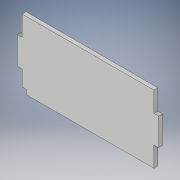
# Autodesk Inventor part: lower_front_wall
Saved by Autodesk Inventor 2018 (Build 220112000, 112)
## iProperties
Created: 2018-04-09
Part Number: lower_front_wall
Material: Generic
Document SubType Name: Modeling
Designer: guita
Density: 1 g/cm^3
Appearance: Default
Author: guita
Autodesk Inventor part; units mm, degrees
ref_plane "YZ Plane" through (0, 0, 0) normal (1, 0, 0) x (0, 1, 0)
ref_plane "XZ Plane" through (0, 0, 0) normal (0, 1, 0) x (-1, 0, 0)
ref_plane "XY Plane" through (0, 0, 0) normal (0, 0, 1) x (1, 0, 0)
sketch "Sketch1" plane through (0, 0, 0) normal (0, 0, 1) x (1, 0, 0)
  line L0 (0, 0) -> (184.15, 0)
  line L1 (184.15, 94.488) -> (0, 94.488)
  line L2 (190.5, 47.244) -> (190.5, 66.294)
  line L3 (190.5, 66.294) -> (184.15, 66.294)
  line L4 (190.5, 47.244) -> (190.5, 28.194)
  line L5 (190.5, 28.194) -> (184.15, 28.194)
  line L6 (-6.35, 47.244) -> (-6.35, 66.294)
  line L7 (-6.35, 66.294) -> (0, 66.294)
  line L8 (-6.35, 47.244) -> (-6.35, 28.194)
  line L9 (-6.35, 28.194) -> (0, 28.194)
  line L10 (0, 94.488) -> (0, 66.294)
  line L11 (0, 28.194) -> (0, 0)
  line L12 (184.15, 0) -> (184.15, 28.194)
  line L13 (184.15, 66.294) -> (184.15, 94.488)
  dimension "d0" = 184.15
  constraints: 28 end point, 11 perpendicular, 5 parallel, 1 horizontal, 1 point on line
  measures "d0" distance of L1.end L1.start
extrude "Extrusion1" add sketch "Sketch1" along normal blind 5.5563
sketch "Sketch2" plane through (0, 0, 0) normal (0, 0, -1) x (-1, 0, 0)
  line L0 (0, 0) -> (0, 6.35)
  line L1 (0, 28.194) -> (0, 0) projected
  line L2 (0, 6.35) -> (-6.35, 6.35)
  line L3 (-6.35, 6.35) -> (-6.35, 0)
  line L4 (0, 6.35) -> (0, 0)
  line L5 (0, 0) -> (-184.15, 0) projected
  line L6 (-6.35, 0) -> (0, 0)
  constraints: 10 end point, 2 collinear, 1 horizontal, 1 perpendicular, 1 point on line
extrude "Extrusion2" cut sketch "Sketch2" against normal blind 6.35
body "Solid1"
